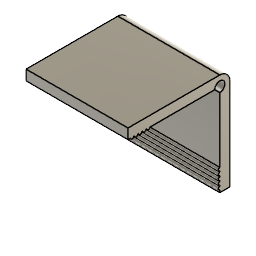
edge piece ridges (Autodesk Fusion 360 design; units mm, degrees)
Autodesk Fusion 360 part; units mm, degrees
note: some values were not read from the file. Set by a fixed rule: which sketch regions a step uses.
sketch "Sketch1" plane through (0, 0, 0) normal (1, 0, 0) x (0, 1, 0)
  line L0 (0, 0) -> (-166.0515, 0)
  line L1 (-166.0515, 0) -> (-166.0515, -106.0261)
  line L2 (-166.0515, -106.0261) -> (0, -106.0261)
  line L3 (0, -106.0261) -> (0, 0)
  line L4 (-90, 0) -> (-90, 10)
  line L5 (-90, 10) -> (0, 10)
  line L6 (10, 0) -> (10, -90)
  line L7 (10, -90) -> (0, -90)
  circle A0 centre (0, 0) radius 5
  arc A1 (10, 0) -> (0, 10) centre (0, 0) ccw
  circle A2 centre (-70, 0) radius 1.5
  circle A3 centre (-74, 0) radius 1.5
  circle A4 centre (-78, 0) radius 1.5
  circle A5 centre (-82, 0) radius 1.5
  circle A6 centre (-86, 0) radius 1.5
  line L8 (-86, 0) -> (-82, 0)
  line L9 (-86, 0) -> (-90, 0)
  line L10 (-82, 0) -> (-78, 0)
  line L11 (-78, 0) -> (-74, 0)
  line L12 (-74, 0) -> (-70, 0)
  line L13 (0, 0) -> (7.0711, 7.0711)
  circle A7 centre (0, -86) radius 1.5
  circle A8 centre (0, -82) radius 1.5
  circle A9 centre (0, -78) radius 1.5
  circle A10 centre (0, -74) radius 1.5
  circle A11 centre (0, -70) radius 1.5
  point P0 (10, 10)
  point P1 (-65.366, 0)
  dimension "d1" = 10
  dimension "d2" = 100
  dimension "d5" = 10
  dimension "d6" = 10
  dimension "d7" = 3
  dimension "d8" = 4
  constraint horizontal L0
  constraint vertical L1
  constraint horizontal L2
  constraint vertical L3
  constraint coincident L0.start L3.end
  constraint coincident L0 L4.start
  constraint perpendicular L0 L4
  constraint perpendicular L4 L5
  constraint perpendicular L0 L6
  constraint coincident L3 L7.end
  constraint perpendicular L3 L7
  constraint equal L4 L7
  constraint coincident P0 L5
  constraint coincident P0 L6
  constraint tangent L5 A1
  constraint tangent L6 A1
  constraint coincident L0 A2.centre
  constraint coincident L0 A3.centre
  constraint coincident L0 A4.centre
  constraint coincident L0 A5.centre
  constraint coincident L0 A6.centre
  constraint equal A2 A3
  constraint equal A4 A5
  constraint equal A5 A6
  constraint equal A3 A4
  constraint coincident A6.centre L8.start
  constraint coincident A5.centre L8.end
  constraint coincident A4.centre L10.end
  constraint coincident A3.centre L11.end
  constraint coincident A2.centre L12.end
  constraint equal L8 L9
  constraint equal L8 L10
  constraint equal L8 L11
  constraint equal L11 L12
  constraint equal L5 L6
  constraint midpoint A1 L13.end
  constraint symmetric A2 L13 A11
  constraint symmetric A3 L13 A10
  constraint symmetric A4 L13 A9
  constraint symmetric A5 L13 A8
  constraint symmetric A6 L13 A7
  measures "d1" distance of L6.end L7.end
  measures "d2" distance of P0 L6.end
  measures "d5" diameter of A0
  measures "d6" radius of A1
  measures "d7" diameter of A4
  measures "d8" distance of L4.start A6.centre
extrude "Extrude1" add sketch "Sketch1" along normal blind 100 contours L0 A2 L12 | L0 L4 L5 A0 A1 A2 A3 A4 A5 A6 L8 L9 L10 L11 L12 L13 | L0 A2 L12 | L3 L6 L7 A0 A1 L13 A7 A8 A9 A10 A11 | L0 A3 L11 L12 | L0 A3 L11 L12 | L3 A11 | L3 A11 | L0 A4 L10 L11 | L0 A4 L10 L11 | L3 A10 | L3 A10 | L0 A5 L8 L10 | L0 A5 L8 L10 | L3 A7 | L3 A7 | L0 A6 L8 L9 | L0 A6 L8 L9 | L3 A9 | L3 A9 | L3 A8 | L3 A8
